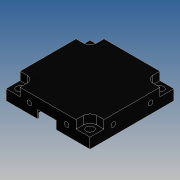
# Autodesk Inventor part: P106
Saved by Autodesk Inventor 2019 (Build 230136000, 136)
## iProperties
Created: 2016-10-19
Part Number: P106
Material: ABS Plastic
Document SubType Name: Modeling
Designer: serge.amoos
Density: 1.06 g/cm^3
Appearance: Smooth - Black
Description: Boîtier de caméra arrière
Author: serge.amoos
Autodesk Inventor part; units mm, degrees
ref_plane "YZ Plane" through (0, 0, 0) normal (1, 0, 0) x (0, 1, 0)
ref_plane "XZ Plane" through (0, 0, 0) normal (0, 1, 0) x (-1, 0, 0)
sketch "Sketch1" plane through (0, 0, 0) normal (0, 0, 1) x (1, 0, 0)
  line L0 (-21.6, 0) -> (3.6, 0) construction
  line L1 (0, -3.6) -> (0, 21.6) construction
  line L2 (-18, 18) -> (0, 18)
  line L3 (0, 18) -> (0, 0)
  line L4 (0, 0) -> (-18, 0)
  line L5 (-18, 0) -> (-18, 18)
  dimension "d0" = 18
  dimension "d1" = 18
  constraints: 8 end point, 2 parallel, 1 horizontal, 1 perpendicular
  measures "d0" distance of L2.start L2.end
  measures "d1" distance of L4.end L2.start
extrude "Extrusion1" add sketch "Sketch1" along normal blind 8
sketch "Sketch2" plane through (0, 0, 8) normal (0, 0, 1) x (1, 0, 0)
  line L0 (-21.6, 0) -> (3.6, 0) projected
  line L1 (0, -3.6) -> (0, 21.6) projected
  point P0 (0, 0)
  point P1 (-15, 15)
  dimension "d4" = 15
  dimension "d5" = 15
  measures "d4" distance from line of L1 point (-15, 15)
  measures "d5" distance from line of L0 point (-15, 15)
hole "Hole1" at (-15, 15, 8) direction (0, 0, -1) diameter 3.2 end through all
sketch "Sketch3" plane through (0, 0, 8) normal (0, 0, 1) x (1, 0, 0)
  line L0 (-21.6, 0) -> (3.6, 0) construction
  line L1 (0, -3.6) -> (0, 21.6) construction
  line L2 (-18, 18) -> (-18, 0) construction
  line L3 (0, 18) -> (-18, 18) construction
  circle A0 centre (-15, 15) radius 1.6 construction
  arc A1 (-15, 12) -> (-12, 15) centre (-15, 15) ccw
  line L4 (-15, 12) -> (-18, 12)
  line L5 (-12, 15) -> (-12, 18)
  line L6 (-12, 18) -> (-18, 18)
  line L7 (-18, 12) -> (-18, 18)
  point P0 (0, 0)
  dimension "d13" = 3
  constraints: 8 end point, 2 collinear, 2 perpendicular, 2 point on circle, 2 point on line, 2 tangent, 1 centre point, 1 coincident
  measures "d13" radius of A1
extrude "Extrusion2" cut sketch "Sketch3" against normal blind 3.5
sketch "Sketch4" plane through (0, 0, 0) normal (0, 0, -1) x (-1, 0, 0)
  line L0 (21.6, 0) -> (-3.6, 0) construction
  line L1 (0, -3.6) -> (0, 21.6) construction
  line L2 (18, 18) -> (18, 0) construction
  line L3 (0, 18) -> (18, 18) construction
  line L4 (17.5, 0) -> (17.5, 12)
  circle A0 centre (15, 15) radius 1.6 construction
  line L5 (17.5, 12) -> (15, 12)
  arc A1 (12, 15) -> (15, 12) centre (15, 15) ccw
  line L6 (12, 15) -> (12, 17.5)
  line L7 (12, 17.5) -> (0, 17.5)
  line L8 (0, 17.5) -> (0, 0)
  line L9 (0, 0) -> (17.5, 0)
  dimension "d19" = 0.5
  dimension "d20" = 0.5
  dimension "d21" = 3
  constraints: 12 end point, 2 collinear, 2 point on circle, 2 point on line, 2 tangent, 2 vertical, 1 centre point, 1 coincident, 1 horizontal, 1 perpendicular
  measures "d19" distance between parallel lines of L4 L2
  measures "d20" distance between parallel lines of L3 L7
  measures "d21" radius of A1
extrude "Extrusion3" cut sketch "Sketch4" against normal blind 2
sketch "Sketch5" plane through (-18, 18, 0) normal (0, 1, 0) x (1, 0, 0)
  line L0 (-3.6, 0) -> (21.6, 0) projected
  line L1 (18, 1.6) -> (18, -9.6) projected
  line L2 (18, -8) -> (6, -8) projected
  point P0 (18, 0)
  point P1 (10, -4.2)
  dimension "d24" = 8
  dimension "d25" = 3.8
  measures "d24" distance from line of L1 point (10, -4.2)
  measures "d25" distance from line of L2 point (10, -4.2)
hole "M3/6/10" at (-8, 18, 4.2) direction (0, -1, 0) diameter 2 depth 2
ref_plane "Work Plane1" through (-18, 18, 0) normal (0.7071, 0.7071, 0) x (0, 0, 1)
mirror "Mirror1" about plane through (-18, 18, 0) normal (0.7071, 0.7071, 0) of "M3/6/10"
pattern_circular "Circular Pattern1" count 4 over 360 about axis through (0, 0, -10) along (0, 0, 1)
sketch "Sketch7" plane through (0, 0, 0) normal (0, 0, -1) x (-1, 0, 0)
  line L0 (25.2, 0) -> (-25.2, 0) construction
  line L1 (0, -27.6) -> (0, 25.6) construction
  line L2 (18, -18) -> (-18, -18) construction
  line L3 (4.5, -11) -> (-3.5, -11)
  line L4 (-3.5, -11) -> (-3.5, -20)
  line L5 (-3.5, -20) -> (4.5, -20)
  line L6 (4.5, -20) -> (4.5, -11)
  line L7 (0.5, -11) -> (0.5, -20) construction
  line L8 (-18, -18) -> (-18, 18) projected
  point P0 (0, 0)
  dimension "d33" = 9
  dimension "d34" = 8
  dimension "d35" = 2
  dimension "d36" = 18.5
  constraints: 10 end point, 2 midpoint, 2 parallel, 1 horizontal, 1 perpendicular
  measures "d33" distance of L5.end L3.start
  measures "d34" distance of L4.end L5.end
  measures "d35" distance between parallel lines of L5 L2
  measures "d36" distance between parallel lines of L8 L7
extrude "Extrusion4" cut sketch "Sketch7" against normal blind 3.5
equation "\"d5\" = d4"
equation "\"d20\" = d19"
body "Solid1"
